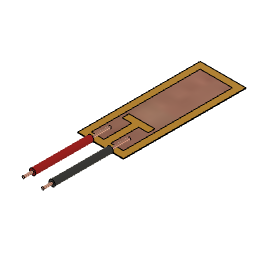
BF350-6AA (Autodesk Fusion 360 design; units mm, degrees)
Autodesk Fusion 360 part; units mm, degrees
note: some values were not read from the file. Set by a fixed rule: which sketch regions a step uses.
sketch "Sketch1" plane through (0, 0, 0) normal (0, 0, 1) x (1, 0, 0)
  line L0 (1.85, -4.95) -> (-1.85, -4.95)
  line L1 (-1.85, -4.95) -> (-1.85, 4.95)
  line L2 (-1.85, 4.95) -> (1.85, 4.95)
  line L3 (1.85, 4.95) -> (1.85, -4.95)
  line L4 (1.85, -4.95) -> (-1.85, 4.95) construction
  line L5 (-1.85, -4.95) -> (1.85, 4.95) construction
  line L6 (-1.3, -1.6) -> (-1.3, 4.4)
  line L7 (-1.3, 4.4) -> (1.3, 4.4)
  line L8 (1.3, 4.4) -> (1.3, -1.6)
  line L9 (1.3, -1.6) -> (-1.3, 4.4) construction
  line L10 (-1.3, -1.6) -> (1.3, 4.4) construction
  line L11 (0, 0) -> (0, 1.4)
  line L12 (-1.3, -1.6) -> (-1.3, -4.4)
  line L13 (-1.3, -4.4) -> (-0.275, -4.4)
  line L14 (-0.275, -4.4) -> (-0.275, -2.15)
  line L15 (-0.275, -2.15) -> (-1.05, -2.15)
  line L16 (-1.05, -2.15) -> (-1.05, -1.6)
  line L17 (1.3, -1.6) -> (1.3, -4.4)
  line L18 (1.3, -4.4) -> (0.275, -4.4)
  line L19 (0.275, -4.4) -> (0.275, -2.15)
  line L20 (0.275, -2.15) -> (1.05, -2.15)
  line L21 (1.05, -2.15) -> (1.05, -1.6)
  line L22 (-1.05, -1.6) -> (1.05, -1.6)
  line L23 (-0.7875, -10.4) -> (-0.8884, -10.4)
  line L24 (-0.8884, -10.4) -> (-0.8884, -4.4)
  line L25 (-0.7875, -4.4) -> (-0.7875, -10.4)
  line L26 (-0.7875, -10.4) -> (-1.0384, -10.4)
  line L27 (-1.0384, -10.4) -> (-1.0384, -4.4)
  line L28 (1.0384, -10.4) -> (1.0384, -4.4)
  line L29 (1.0384, -4.4) -> (0.7875, -4.4)
  line L30 (0.7875, -4.4) -> (0.7875, -10.4)
  line L31 (0.7875, -10.4) -> (1.0384, -10.4)
  line L32 (0.8884, -10.4) -> (0.8884, -4.4)
  line L33 (-1.0384, -9.65) -> (-0.8884, -9.65)
  line L34 (1.0384, -9.65) -> (0.8884, -9.65)
  line L35 (-0.8884, -4.4) -> (-0.8884, -3.4)
  line L36 (-0.7875, -3.4) -> (-0.7875, -4.4)
  line L37 (-0.7875, -3.4) -> (-0.8884, -3.4)
  line L38 (0.8884, -4.4) -> (0.8884, -3.4)
  line L39 (0.7875, -3.4) -> (0.8884, -3.4)
  line L40 (0.7875, -3.4) -> (0.7875, -4.4)
  point P0 (0, 1.4)
  dimension "d3" = 3.7
  dimension "d4" = 9.9
  dimension "d5" = 2.6
  dimension "d7" = 0.55
  dimension "d8" = 0.55
  dimension "d9" = 0.55
  dimension "d13" = 0.25
  dimension "d17" = 0.55
  dimension "d20" = 0.55
  dimension "d21" = 6
  dimension "d22" = 0.55
  dimension "d27" = 0.1009
  dimension "d28" = 6
  dimension "d30" = 0.15
  dimension "d33" = 0.75
  dimension "d36" = 1
  constraint coincident L11.start origin
  constraint horizontal L0
  constraint perpendicular L0 L1
  constraint parallel L0 L2
  constraint parallel L1 L3
  constraint coincident L4 L11.start
  constraint coincident L5 L11.start
  constraint parallel L6 L8
  constraint coincident L9 P0
  constraint coincident L10 P0
  constraint vertical L11
  constraint coincident P0 L11.end
  constraint perpendicular L12 L13
  constraint perpendicular L13 L14
  constraint perpendicular L14 L15
  constraint symmetric L6.start L11 L8.end
  constraint symmetric L11 L12.end L17.end
  constraint symmetric L11 L13.end L18.end
  constraint symmetric L11 L14.end L19.end
  constraint symmetric L11 L15.end L20.end
  constraint symmetric L11 L16.end L21.end
  constraint horizontal L23
  constraint vertical L24
  constraint vertical L25
  constraint horizontal L26
  constraint vertical L27
  constraint coincident L23.start L25
  constraint coincident L36.end L25
  constraint coincident L23.end L26
  constraint midpoint L13 L25.start
  constraint symmetric L11 L24.end L32.end
  constraint symmetric L11 L23.end L32.start
  constraint symmetric L11 L27.end L28.end
  constraint symmetric L11 L25.start L29.end
  constraint symmetric L11 L23.start L30.end
  constraint symmetric L11 L26.end L28.start
  constraint coincident L27 L33.start
  constraint coincident L24 L33.end
  constraint perpendicular L24 L33
  constraint symmetric L11 L33.start L34.start
  constraint symmetric L11 L33.end L34.end
  constraint perpendicular L13 L36
  constraint perpendicular L35 L37
  constraint symmetric L11 L35.end L38.end
  constraint symmetric L11 L36.start L39.start
  constraint coincident L35.end L37.end
  constraint coincident L13 L27.end
  constraint vertical L8
  constraint coincident L6.start L22
  constraint coincident L8.end L9.start
  constraint coincident L25.start L36.end
  constraint coincident L13 L24.end
  constraint vertical L35
  measures "d3" distance of L1.end L2.end
  measures "d4" distance of L0.end L1.end
  measures "d5" distance of L6.end L7.end
  measures "d7" distance of L2 L7
  measures "d8" distance of L3 L8
  measures "d9" distance of L1 L6
  measures "d13" distance of L12 L16
  measures "d17" distance of L0 L13
  measures "d20" distance of L15 L22
  measures "d21" distance of L7 L22
  measures "d22" distance of L14 L19
  measures "d27" distance of L24.end L25.start
  measures "d28" distance of L24.end L23.end
  measures "d30" distance of L24 L27
  measures "d33" distance of L26 L33
  measures "d36" vertical distance of L24.end L35.end
extrude "Extrude1" add sketch "Sketch1" against normal blind 0.05 contours L0 L1 L2 L3 L6 L7 L8 L12 L13 L17 L18 L27 L28 | L0 L18 L28 L29 L32 | L0 L18 L29 L30 L32 | L6 L7 L8 L12 L13 L14 L15 L16 L17 L18 L19 L20 L21 L22 L29 L35 L36 L37 L38 L39 L40 | L0 L13 L14 L15 L16 L18 L19 L20 L21 L22 L25 L30 | L18 L29 L38 L39 L40 | L0 L13 L24 L25 | L0 L13 L24 L27 | L13 L35 L36 L37 makes body 1
extrude "Extrude2" add sketch "Sketch1" along normal blind 0.005 separate body contours L6 L7 L8 L12 L13 L14 L15 L16 L17 L18 L19 L20 L21 L22 L29 L35 L36 L37 L38 L39 L40 | L18 L29 L38 L39 L40 | L13 L35 L36 L37 makes body 2
revolve "Revolve1" add sketch "Sketch1" angle 360 about axis through (-0.7875, -4.4, 0) along (0, -1, 0) separate body contours L0 L23 L24 L25 L26 | L0 L13 L24 L25 | L13 L35 L36 L37 makes body 3
revolve "Revolve2" add sketch "Sketch1" angle 360 about axis through (-0.7875, -4.4, 0) along (0, -1, 0) separate body contours L0 L24 L27 L33 makes body 4
revolve "Revolve3" add sketch "Sketch1" angle 360 about axis through (0.7875, -4.4, 0) along (0, -1, 0) separate body contours L0 L30 L31 L32 | L0 L18 L29 L30 L32 | L18 L29 L38 L39 L40 makes body 5
revolve "Revolve4" add sketch "Sketch1" angle 360 about axis through (0.7875, -4.4, 0) along (0, -1, 0) separate body contours L0 L28 L32 L34 makes body 6
move_body "Move1" bodies 6 4 5 3 to x (1, 0, 0) y (0, 1, 0) z (0, 0, 1) at (0, 0, 0.101)
equation "d27 = ( 0.2019 / 2 ) * 1 mm"
